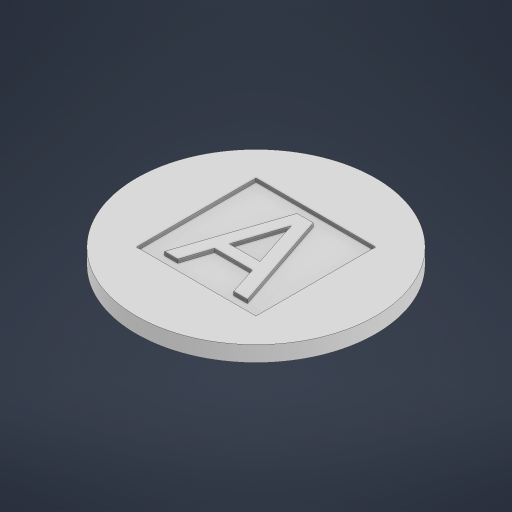
# Autodesk Inventor part: TopMarkerPreset
Saved by Autodesk Inventor 2023.2 (Build 272271030, 271C)
## iProperties
Created: 2023-05-05
Part Number: TopMarkerPreset
Material: Generic
Document SubType Name: Modeling
Designer: Elias Braun
Density: 1 g/cm^3
Appearance: Default
Author: Elias Braun
Autodesk Inventor part; units mm, degrees
ref_plane "YZ Plane" through (0, 0, 0) normal (1, 0, 0) x (0, 1, 0)
ref_plane "XZ Plane" through (0, 0, 0) normal (0, 1, 0) x (-1, 0, 0)
ref_plane "XY Plane" through (0, 0, 0) normal (0, 0, 1) x (1, 0, 0)
sketch "Sketch1" plane through (0, 0, 0) normal (0, 1, 0) x (-1, 0, 0)
  circle A0 centre (0, 0) radius 20
  dimension "d0" = 40
  constraints: 1 centre point, 1 coincident
  measures "d0" diameter of A0
extrude "Extrusion1" add sketch "Sketch1" along normal blind 2.6
sketch "Sketch2" plane through (0, 2.6, 0) normal (0, 1, 0) x (1, 0, 0)
  line L0 (-10, -10) -> (-10, 10)
  line L1 (-10, 10) -> (10, 10)
  line L2 (10, 10) -> (10, -10)
  line L3 (10, -10) -> (-10, -10)
  line L4 (-10, -10) -> (10, 10) construction
  line L5 (-10, 10) -> (10, -10) construction
  point P0 (0, 0)
  dimension "d3" = 20
  dimension "d4" = 20
  constraints: 12 end point, 2 midpoint, 2 parallel, 1 perpendicular, 1 vertical
  measures "d3" distance of L0.start L0.end
  measures "d4" distance of L0.end L1.end
extrude "Extrusion2" cut sketch "Sketch2" against normal blind 0.6
sketch "Sketch3" plane through (0, 2, 0) normal (0, 1, 0) x (1, 0, 0)
  line L0 (-6.9184, 8.3) -> (6.9911, 8.3) construction
  line L1 (6.9911, 8.3) -> (6.9911, -8.3) construction
  line L2 (6.9911, -8.3) -> (-6.9184, -8.3) construction
  line L3 (-6.9184, -8.3) -> (-6.9184, 8.3) construction
  line L4 (-7.026, -8.3) -> (-1.4299, 8.3)
  line L5 (-1.4299, 8.3) -> (1.2874, 8.3)
  line L6 (1.2874, 8.3) -> (6.8835, -8.3)
  line L7 (6.8835, -8.3) -> (4.5563, -8.3)
  line L8 (4.5563, -8.3) -> (3.0496, -3.659)
  line L9 (3.0496, -3.659) -> (-3.2863, -3.659)
  line L10 (-3.2863, -3.659) -> (-4.793, -8.3)
  line L11 (-4.793, -8.3) -> (-7.026, -8.3)
  line L12 (2.4443, -1.7757) -> (-0.1251, 6.04)
  line L13 (-0.1251, 6.04) -> (-2.681, -1.7757)
  line L14 (-2.681, -1.7757) -> (2.4443, -1.7757)
  point P0 (0, 0)
  constraints: 2 other
extrude "Extrusion3" add sketch "Sketch3" along normal blind 0.6
body "Solid1"
